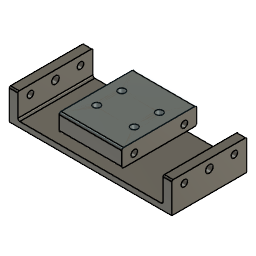
Sample Fixtures (Autodesk Fusion 360 archive; units mm, degrees)
design "Updated X stage"
part number: 2026-06-25-14-53-23-584
Autodesk Fusion 360 part; units mm, degrees
sketch "Sketch1" plane through (0, 0, 0) normal (0, 0, 1) x (1, 0, 0)
  line L0 (65, -30) -> (-65, -30)
  line L1 (-65, -30) -> (-65, 30)
  line L2 (-65, 30) -> (65, 30)
  line L3 (65, 30) -> (65, -30)
  line L4 (65, -30) -> (-65, 30) construction
  line L5 (-65, -30) -> (65, 30) construction
  line L6 (10, -15) -> (-10, -15) construction
  line L7 (-10, -15) -> (-10, 15) construction
  line L8 (-10, 15) -> (10, 15) construction
  line L9 (10, 15) -> (10, -15) construction
  line L10 (10, -15) -> (-10, 15) construction
  line L11 (-10, -15) -> (10, 15) construction
  circle A0 centre (10, 15) radius 2.05
  circle A1 centre (10, -15) radius 2.05
  circle A2 centre (-10, -15) radius 2.05
  circle A3 centre (-10, 15) radius 2.05
  dimension "d1" = 60
  dimension "d2" = 130
  dimension "d5" = 20
  dimension "d6" = 30
  dimension "d7" = 4.1
  constraint horizontal L0
  constraint perpendicular L0 L1
  constraint parallel L0 L2
  constraint parallel L1 L3
  constraint coincident L4 origin
  constraint coincident L5 origin
  constraint horizontal L6
  constraint perpendicular L6 L7
  constraint parallel L6 L8
  constraint parallel L7 L9
  constraint coincident L10 origin
  constraint coincident L11 origin
  constraint coincident L8.end L9.start
  constraint coincident L6.start L9.end
  constraint coincident L6.end L7.start
  constraint coincident L7.end L8.start
  constraint equal A0 A1
  constraint equal A1 A2
  constraint equal A2 A3
  measures "d1" distance of L0.start L2.end
  measures "d2" distance of L1.end L2.end
  measures "d5" distance of L7.end L8.end
  measures "d6" distance of L6.start L8.end
  measures "d7" diameter of A0
extrude "Extrude1" add sketch "Sketch1" along normal blind 4.5 makes body 1
sketch "Sketch2" plane through (0, 0, 4.5) normal (0, 0, 1) x (-1, 0, 0)
  circle A0 centre (10, 15) radius 2.05
  circle A1 centre (-10, 15) radius 2.05
  circle A2 centre (-10, -15) radius 2.05
  circle A3 centre (10, -15) radius 2.05
  line L0 (-65, -30) -> (65, -30)
  line L1 (65, -30) -> (65, 30)
  line L2 (65, 30) -> (-65, 30)
  line L3 (-65, 30) -> (-65, -30)
  line L4 (-10, 15) -> (10, 15) construction
  line L5 (10, 15) -> (10, -15) construction
  line L6 (10, -15) -> (-10, -15) construction
  line L7 (-10, -15) -> (-10, 15) construction
  line L8 (-10, 15) -> (10, -15) construction
  line L9 (10, 15) -> (-10, -15) construction
  circle A4 centre (-10, -15) radius 3.65
  circle A5 centre (-10, 15) radius 3.65
  circle A6 centre (10, 15) radius 3.65
  circle A7 centre (10, -15) radius 3.65
  dimension "d8" = 7.3
  constraint horizontal L4
  constraint perpendicular L4 L5
  constraint parallel L4 L6
  constraint parallel L5 L7
  constraint coincident L8 origin
  constraint coincident L9 origin
  constraint coincident A1.centre L4.start
  constraint concentric A2 A4
  constraint concentric A0 A6
  constraint concentric A3 A7
  constraint equal A4 A5
  constraint equal A5 A6
  constraint equal A6 A7
  measures "d8" diameter of A4
  measures "d27" diameter of origin
extrude "Extrude2" cut sketch "Sketch2" against normal blind 3.2 contours A4 | A5 | A6 | A7 bodies 1
sketch "Sketch3" plane through (0, 0, 4.5) normal (0, 0, 1) x (-1, 0, 0)
  line L0 (-65, -30) -> (65, -30)
  line L1 (65, -30) -> (65, 30)
  line L2 (65, 30) -> (-65, 30)
  line L3 (-65, 30) -> (-65, -30)
  circle A0 centre (10, -15) radius 3.65
  circle A1 centre (-10, -15) radius 3.65
  circle A2 centre (10, 15) radius 3.65
  circle A3 centre (-10, 15) radius 3.65
  line L4 (65, -30) -> (58, -30)
  line L5 (58, -30) -> (58, 30)
  line L6 (58, 30) -> (65, 30)
  line L7 (65, 30) -> (65, -30)
  line L8 (-65, -30) -> (-58, -30)
  line L9 (-58, -30) -> (-58, 30)
  line L10 (-58, 30) -> (-65, 30)
  line L11 (-65, 30) -> (-65, -30)
  dimension "d11" = 7
  dimension "d12" = 7
  constraint horizontal L4
  constraint vertical L5
  constraint horizontal L6
  constraint vertical L7
  constraint coincident L2 L5.end
  constraint coincident L0.end L1.start
  constraint horizontal L8
  constraint vertical L9
  constraint horizontal L10
  constraint vertical L11
  constraint coincident L2 L9.end
  constraint coincident L0.start L3.end
  measures "d11" distance of L5 L7
  measures "d12" distance of L9 L11
extrude "Extrude3" add sketch "Sketch3" along normal blind 20 contours L0 L2 L3 L8 L9 L10 L11 | L0 L1 L2 L4 L5 L6 L7 bodies 1
sketch "Sketch4" plane through (65, 0, 0) normal (1, 0, 0) x (0, 1, 0)
  line L0 (-30, 0) -> (30, 0)
  line L1 (30, 0) -> (30, 24.5)
  line L2 (30, 24.5) -> (-30, 24.5)
  line L3 (-30, 24.5) -> (-30, 0)
  line L4 (-30.1781, 17.5) -> (30.1781, 17.5) construction
  circle A0 centre (-20, 17.5) radius 2.575
  circle A1 centre (0, 17.5) radius 3
  circle A2 centre (20, 17.5) radius 2.575
  line L5 (30, 0) -> (-30, 0)
  line L6 (0, 24.5) -> (0, 0) construction
  dimension "d15" = 6
  dimension "d16" = 20
  dimension "d17" = 20
  dimension "d36" = 7
  dimension "d48" = 5.15
  constraint coincident L4 A0.centre
  constraint midpoint L4 A1.centre
  constraint coincident L4 A2.centre
  constraint midpoint L2 L6.start
  constraint coincident L6.end origin
  constraint coincident A1.centre L6
  constraint equal A0 A2
  measures "d15" diameter of A1
  measures "d16" distance of A1.centre A2.centre
  measures "d17" distance of A0.centre A1.centre
  measures "d36" distance of L2 L4
  measures "d48" diameter of A2
extrude "Extrude4" cut sketch "Sketch4" against normal through all contours A0 | A1 | A2 bodies 1
ref_plane "WorkPlane1" through (0, 0, 12.5) normal (0, 0, 1) x (1, 0, 0)
sketch "Sketch5" plane through (0, 0, 12.5) normal (0, 0, 1) x (1, 0, 0)
  line L0 (-25, 30) -> (25, 30)
  line L1 (25, 30) -> (25, -30)
  line L2 (25, -30) -> (-25, -30)
  line L3 (-25, -30) -> (-25, 30)
  line L4 (-25, 30) -> (25, -30) construction
  line L5 (25, 30) -> (-25, -30) construction
  line L6 (-65, 30) -> (65, 30)
  dimension "d22" = 50
  constraint horizontal L0
  constraint perpendicular L0 L1
  constraint parallel L0 L2
  constraint parallel L1 L3
  constraint coincident L4 origin
  constraint coincident L5 origin
  constraint collinear L0 L6
  measures "d22" distance of L1.end L2.end
extrude "Extrude5" add sketch "Sketch5" along normal blind 14 separate body makes body 2
sketch "Sketch6" plane through (0, 0, 26.5) normal (0, 0, 1) x (-1, 0, 0)
  line L0 (25, -30) -> (25, 30)
  line L1 (25, 30) -> (-25, 30)
  line L2 (-25, 30) -> (-25, -30)
  line L3 (-25, -30) -> (25, -30)
  line L4 (15, -10) -> (-15, -10) construction
  line L5 (-15, -10) -> (-15, 10) construction
  line L6 (-15, 10) -> (15, 10) construction
  line L7 (15, 10) -> (15, -10) construction
  line L8 (15, -10) -> (-15, 10) construction
  line L9 (-15, -10) -> (15, 10) construction
  circle A0 centre (-15, 10) radius 2.8
  circle A1 centre (15, 10) radius 2.8
  circle A2 centre (15, -10) radius 2.8
  circle A3 centre (-15, -10) radius 2.8
  dimension "d25" = 20
  dimension "d26" = 30
  dimension "d27" = 5.6
  constraint horizontal L4
  constraint perpendicular L4 L5
  constraint parallel L4 L6
  constraint parallel L5 L7
  constraint coincident L8 origin
  constraint coincident L9 origin
  constraint coincident L5.end L6.start
  constraint coincident L6.end L7.start
  constraint coincident L4.start L7.end
  constraint coincident L4.end L5.start
  constraint equal A0 A3
  constraint equal A0 A1
  constraint equal A1 A2
  measures "d25" distance of L4.end L5.end
  measures "d26" distance of L5.end L6.end
  measures "d27" diameter of A3
extrude "Extrude6" cut sketch "Sketch6" against normal up to surface (14 mm away) contours A0 | A1 | A2 | A3 bodies 2
sketch "Sketch7" plane through (25, 0, 0) normal (1, 0, 0) x (0, 1, 0)
  line L0 (30, 26.5) -> (-30, 26.5)
  line L1 (-30, 26.5) -> (-30, 12.5)
  line L2 (-30, 12.5) -> (30, 12.5)
  line L3 (30, 12.5) -> (30, 26.5)
  line L4 (-30, 18.3) -> (30, 18.3) construction
  circle A0 centre (-20, 18.3) radius 2.6
  circle A1 centre (0, 18.3) radius 3
  circle A2 centre (20, 18.3) radius 2.6
  dimension "d30" = 8.2
  dimension "d31" = 20
  dimension "d32" = 20
  dimension "d33" = 6
  dimension "d49" = 5.2
  constraint coincident L1 L4.start
  constraint coincident L3 L4.end
  constraint perpendicular L3 L4
  constraint coincident L4 A0.centre
  constraint midpoint L4 A1.centre
  constraint coincident L4 A2.centre
  constraint equal A0 A2
  measures "d30" distance of L0 L4
  measures "d31" distance of A1.centre A2.centre
  measures "d32" distance of A0.centre A1.centre
  measures "d33" diameter of A1
  measures "d49" diameter of A0
extrude "Extrude7" cut sketch "Sketch7" against normal up to surface (50 mm away) contours A0 | A2 bodies 2
sketch "Sketch8" plane through (65, 0, 0) normal (1, 0, 0) x (0, 1, 0)
  circle A0 centre (20, 17.5) radius 2.575
  circle A1 centre (-20, 17.5) radius 2.575
  circle A2 centre (0, 17.5) radius 3
  line L0 (-30, 0) -> (30, 0)
  line L1 (30, 0) -> (30, 24.5)
  line L2 (30, 24.5) -> (-30, 24.5)
  line L3 (-30, 24.5) -> (-30, 0)
  circle A3 centre (-20, 17.5) radius 2.95
  circle A4 centre (20, 17.5) radius 2.95
  dimension "d38" = 5.9
  constraint coincident A1.centre A3.centre
  constraint coincident A0.centre A4.centre
  constraint equal A3 A4
  measures "d38" diameter of A4
extrude "Extrude8" add sketch "Sketch8" against normal up to surface (130 mm away) separate body contours A0 | A1 | A3 | A4 makes body 3 at (21.6667, 22.9353, 17.2063) makes body 4 at (-21.6667, -17.0537, 17.353)
sketch "Sketch9" plane through (0, 0, 26.5) normal (0, 0, 1) x (-1, 0, 0)
  circle A0 centre (-15, -10) radius 2.8
  circle A1 centre (15, -10) radius 2.8
  circle A2 centre (-15, 10) radius 2.8
  circle A3 centre (15, 10) radius 2.8
  line L0 (25, 30) -> (-25, 30)
  line L1 (-25, 30) -> (-25, -30)
  line L2 (-25, -30) -> (25, -30)
  line L3 (25, -30) -> (25, 30)
split "Split1" by plane through (0, 0, 0) normal (1, 0, 0) bodies 3 makes body 5 at (21.6667, 22.9353, 17.2063)
sketch "Sketch10" plane through (0, 0, 0) normal (1, 0, 0) x (0, 1, 0)
  circle A0 centre (20, 17.5) radius 2.95
  circle A1 centre (20, 17.5) radius 1.25
  dimension "d42" = 2.5
  constraint concentric A0 A1
  measures "d42" diameter of A1
extrude "Extrude9" add sketch "Sketch10" along normal blind 4 contours A1 bodies 3
sketch "Sketch11" plane through (0, 0, 0) normal (-1, 0, 0) x (0, -1, 0)
  circle A0 centre (-20, 17.5) radius 2.95
  circle A1 centre (-20, 17.5) radius 1.325
  dimension "d45" = 2.65
  constraint concentric A0 A1
  measures "d45" diameter of A1
extrude "Extrude10" cut sketch "Sketch11" against normal blind 4 contours A1 bodies 5
sketch "Sketch12" plane through (0, 0, 0) normal (0, 1, 0) x (1, 0, 0)
fillet "Fillet1" radius 1 4 edges at (-61.5, 30, 24.5) (61.5, 30, 24.5) (61.5, -30, 24.5) (-61.5, -30, 24.5) on bodies 1
fillet "Fillet2" radius 1.5 2 edges at (-58, 0, 4.5) (58, 0, 4.5) on bodies 1
fillet "Fillet3" radius 1.5 2 edges at (0, -30, 12.5) (0, 30, 12.5) on bodies 2
fillet "Fillet3" radius 1.5 2 edges at (0, 30, 26.5) (0, -30, 26.5) on bodies 2
delete_body "RemoveBody1" bodies 3
delete_body "RemoveBody2" bodies 4
delete_body "RemoveBody3" bodies 5
named bodies: "Ystage", "Y mount", "Male Support rod", "Support rod (1)"

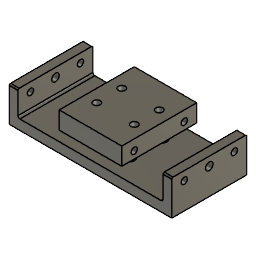
design "Updated Y stage"
part number: 2026-06-25-14-53-23-584
Autodesk Fusion 360 part; units mm, degrees
sketch "Sketch1" plane through (0, 0, 0) normal (0, 0, 1) x (1, 0, 0)
  line L0 (65, -30) -> (-65, -30)
  line L1 (-65, -30) -> (-65, 30)
  line L2 (-65, 30) -> (65, 30)
  line L3 (65, 30) -> (65, -30)
  line L4 (65, -30) -> (-65, 30) construction
  line L5 (-65, -30) -> (65, 30) construction
  line L6 (13, -13) -> (-13, -13) construction
  line L7 (-13, -13) -> (-13, 13) construction
  line L8 (-13, 13) -> (13, 13) construction
  line L9 (13, 13) -> (13, -13) construction
  line L10 (13, -13) -> (-13, 13) construction
  line L11 (-13, -13) -> (13, 13) construction
  circle A0 centre (13, 13) radius 3
  circle A1 centre (13, -13) radius 3
  circle A2 centre (-13, -13) radius 3
  circle A3 centre (-13, 13) radius 3
  dimension "d1" = 60
  dimension "d2" = 130
  dimension "d5" = 26
  dimension "d6" = 26
  dimension "d7" = 6
  constraint horizontal L0
  constraint perpendicular L0 L1
  constraint parallel L0 L2
  constraint parallel L1 L3
  constraint coincident L4 origin
  constraint coincident L5 origin
  constraint horizontal L6
  constraint perpendicular L6 L7
  constraint parallel L6 L8
  constraint parallel L7 L9
  constraint coincident L10 origin
  constraint coincident L11 origin
  constraint coincident L8.end L9.start
  constraint coincident L6.start L9.end
  constraint coincident L6.end L7.start
  constraint coincident L7.end L8.start
  constraint equal A0 A1
  constraint equal A1 A2
  constraint equal A2 A3
  measures "d1" distance of L0.start L2.end
  measures "d2" distance of L1.end L2.end
  measures "d5" distance of L7.end L8.end
  measures "d6" distance of L6.start L8.end
  measures "d7" diameter of A0
extrude "Extrude1" add sketch "Sketch1" along normal blind 8 makes body 1
sketch "Sketch2" plane through (0, 0, 8) normal (0, 0, 1) x (-1, 0, 0)
  circle A0 centre (13, 13) radius 3
  circle A1 centre (-13, 13) radius 3
  circle A2 centre (-13, -13) radius 3
  circle A3 centre (13, -13) radius 3
  line L0 (-65, -30) -> (65, -30)
  line L1 (65, -30) -> (65, 30)
  line L2 (65, 30) -> (-65, 30)
  line L3 (-65, 30) -> (-65, -30)
  line L4 (-13, 13) -> (13, 13) construction
  line L5 (13, 13) -> (13, -13) construction
  line L6 (13, -13) -> (-13, -13) construction
  line L7 (-13, -13) -> (-13, 13) construction
  line L8 (-13, 13) -> (13, -13) construction
  line L9 (13, 13) -> (-13, -13) construction
  circle A4 centre (-13, -13) radius 5.15
  circle A5 centre (-13, 13) radius 5.15
  circle A6 centre (13, 13) radius 5.15
  circle A7 centre (13, -13) radius 5.15
  dimension "d8" = 10.3
  constraint horizontal L4
  constraint perpendicular L4 L5
  constraint parallel L4 L6
  constraint parallel L5 L7
  constraint coincident L8 origin
  constraint coincident L9 origin
  constraint coincident A1.centre L4.start
  constraint concentric A2 A4
  constraint concentric A0 A6
  constraint concentric A3 A7
  constraint equal A4 A5
  constraint equal A5 A6
  constraint equal A6 A7
  measures "d8" diameter of A4
  measures "d27" diameter of origin
extrude "Extrude2" cut sketch "Sketch2" against normal blind 6.1 contours A4 | A5 | A6 | A7 bodies 1
sketch "Sketch3" plane through (0, 0, 8) normal (0, 0, 1) x (-1, 0, 0)
  line L0 (-65, -30) -> (65, -30)
  line L1 (65, -30) -> (65, 30)
  line L2 (65, 30) -> (-65, 30)
  line L3 (-65, 30) -> (-65, -30)
  circle A0 centre (13, -13) radius 5.15
  circle A1 centre (-13, -13) radius 5.15
  circle A2 centre (13, 13) radius 5.15
  circle A3 centre (-13, 13) radius 5.15
  line L4 (65, -30) -> (58, -30)
  line L5 (58, -30) -> (58, 30)
  line L6 (58, 30) -> (65, 30)
  line L7 (65, 30) -> (65, -30)
  line L8 (-65, -30) -> (-58, -30)
  line L9 (-58, -30) -> (-58, 30)
  line L10 (-58, 30) -> (-65, 30)
  line L11 (-65, 30) -> (-65, -30)
  dimension "d11" = 7
  dimension "d12" = 7
  constraint horizontal L4
  constraint vertical L5
  constraint horizontal L6
  constraint vertical L7
  constraint coincident L2 L5.end
  constraint coincident L0.end L1.start
  constraint horizontal L8
  constraint vertical L9
  constraint horizontal L10
  constraint vertical L11
  constraint coincident L2 L9.end
  constraint coincident L0.start L3.end
  measures "d11" distance of L5 L7
  measures "d12" distance of L9 L11
extrude "Extrude3" add sketch "Sketch3" along normal blind 20 contours L0 L2 L3 L8 L9 L10 L11 | L0 L1 L2 L4 L5 L6 L7 bodies 1
sketch "Sketch4" plane through (65, 0, 0) normal (1, 0, 0) x (0, 1, 0)
  line L0 (-30, 0) -> (30, 0)
  line L1 (30, 0) -> (30, 28)
  line L2 (30, 28) -> (-30, 28)
  line L3 (-30, 28) -> (-30, 0)
  line L4 (-30.1781, 21) -> (30.1781, 21) construction
  circle A0 centre (-20, 21) radius 2.5
  circle A1 centre (0, 21) radius 3
  circle A2 centre (20, 21) radius 2.5
  line L5 (30, 0) -> (-30, 0)
  line L6 (0, 28) -> (0, 0) construction
  dimension "d15" = 6
  dimension "d16" = 20
  dimension "d17" = 20
  dimension "d36" = 7
  dimension "d48" = 5
  constraint coincident L4 A0.centre
  constraint midpoint L4 A1.centre
  constraint coincident L4 A2.centre
  constraint midpoint L2 L6.start
  constraint coincident L6.end origin
  constraint coincident A1.centre L6
  constraint equal A0 A2
  measures "d15" diameter of A1
  measures "d16" distance of A1.centre A2.centre
  measures "d17" distance of A0.centre A1.centre
  measures "d36" distance of L2 L4
  measures "d48" diameter of A2
extrude "Extrude4" cut sketch "Sketch4" against normal through all contours A0 | A1 | A2 bodies 1
ref_plane "WorkPlane1" through (0, 0, 16) normal (0, 0, 1) x (1, 0, 0)
sketch "Sketch5" plane through (0, 0, 16) normal (0, 0, 1) x (1, 0, 0)
  line L0 (-25, 30) -> (25, 30)
  line L1 (25, 30) -> (25, -30)
  line L2 (25, -30) -> (-25, -30)
  line L3 (-25, -30) -> (-25, 30)
  line L4 (-25, 30) -> (25, -30) construction
  line L5 (25, 30) -> (-25, -30) construction
  line L6 (-65, 30) -> (65, 30)
  dimension "d22" = 50
  constraint horizontal L0
  constraint perpendicular L0 L1
  constraint parallel L0 L2
  constraint parallel L1 L3
  constraint coincident L4 origin
  constraint coincident L5 origin
  constraint collinear L0 L6
  measures "d22" distance of L1.end L2.end
extrude "Extrude5" add sketch "Sketch5" along normal blind 14 separate body makes body 2
sketch "Sketch6" plane through (0, 0, 30) normal (0, 0, 1) x (-1, 0, 0)
  line L0 (25, -30) -> (25, 30)
  line L1 (25, 30) -> (-25, 30)
  line L2 (-25, 30) -> (-25, -30)
  line L3 (-25, -30) -> (25, -30)
  line L4 (15, -10) -> (-15, -10) construction
  line L5 (-15, -10) -> (-15, 10) construction
  line L6 (-15, 10) -> (15, 10) construction
  line L7 (15, 10) -> (15, -10) construction
  line L8 (15, -10) -> (-15, 10) construction
  line L9 (-15, -10) -> (15, 10) construction
  circle A0 centre (-15, 10) radius 2.8
  circle A1 centre (15, 10) radius 2.8
  circle A2 centre (15, -10) radius 2.8
  circle A3 centre (-15, -10) radius 2.8
  dimension "d25" = 20
  dimension "d26" = 30
  dimension "d27" = 5.6
  constraint horizontal L4
  constraint perpendicular L4 L5
  constraint parallel L4 L6
  constraint parallel L5 L7
  constraint coincident L8 origin
  constraint coincident L9 origin
  constraint coincident L5.end L6.start
  constraint coincident L6.end L7.start
  constraint coincident L4.start L7.end
  constraint coincident L4.end L5.start
  constraint equal A0 A3
  constraint equal A0 A1
  constraint equal A1 A2
  measures "d25" distance of L4.end L5.end
  measures "d26" distance of L5.end L6.end
  measures "d27" diameter of A3
extrude "Extrude6" cut sketch "Sketch6" against normal up to surface (14 mm away) contours A0 | A1 | A2 | A3 bodies 2
sketch "Sketch7" plane through (25, 0, 0) normal (1, 0, 0) x (0, 1, 0)
  line L0 (30, 30) -> (-30, 30)
  line L1 (-30, 30) -> (-30, 16)
  line L2 (-30, 16) -> (30, 16)
  line L3 (30, 16) -> (30, 30)
  line L4 (-30, 21.8) -> (30, 21.8) construction
  circle A0 centre (-20, 21.8) radius 2.5
  circle A1 centre (0, 21.8) radius 3
  circle A2 centre (20, 21.8) radius 2.5
  dimension "d30" = 8.2
  dimension "d31" = 20
  dimension "d32" = 20
  dimension "d33" = 6
  dimension "d49" = 5
  constraint coincident L1 L4.start
  constraint coincident L3 L4.end
  constraint perpendicular L3 L4
  constraint coincident L4 A0.centre
  constraint midpoint L4 A1.centre
  constraint coincident L4 A2.centre
  constraint equal A0 A2
  measures "d30" distance of L0 L4
  measures "d31" distance of A1.centre A2.centre
  measures "d32" distance of A0.centre A1.centre
  measures "d33" diameter of A1
  measures "d49" diameter of A0
extrude "Extrude7" cut sketch "Sketch7" against normal up to surface (50 mm away) contours A0 | A2 bodies 2
sketch "Sketch8" plane through (65, 0, 0) normal (1, 0, 0) x (0, 1, 0)
  circle A0 centre (20, 21) radius 2.5
  circle A1 centre (-20, 21) radius 2.5
  circle A2 centre (0, 21) radius 3
  line L0 (-30, 0) -> (30, 0)
  line L1 (30, 0) -> (30, 28)
  line L2 (30, 28) -> (-30, 28)
  line L3 (-30, 28) -> (-30, 0)
  circle A3 centre (-20, 21) radius 2.95
  circle A4 centre (20, 21) radius 2.95
  dimension "d38" = 5.9
  constraint coincident A1.centre A3.centre
  constraint coincident A0.centre A4.centre
  constraint equal A3 A4
  measures "d38" diameter of A4
extrude "Extrude8" add sketch "Sketch8" against normal up to surface (130 mm away) separate body contours A0 | A1 | A3 | A4 makes body 3 at (21.6667, 22.9353, 20.7063) makes body 4 at (-21.6667, -17.0537, 20.853)
sketch "Sketch9" plane through (0, 0, 30) normal (0, 0, 1) x (-1, 0, 0)
  circle A0 centre (-15, -10) radius 2.8
  circle A1 centre (15, -10) radius 2.8
  circle A2 centre (-15, 10) radius 2.8
  circle A3 centre (15, 10) radius 2.8
  line L0 (25, 30) -> (-25, 30)
  line L1 (-25, 30) -> (-25, -30)
  line L2 (-25, -30) -> (25, -30)
  line L3 (25, -30) -> (25, 30)
split "Split1" by plane through (0, 0, 0) normal (1, 0, 0) bodies 3 makes body 5 at (21.6667, 22.9353, 20.7063)
sketch "Sketch10" plane through (0, 0, 0) normal (1, 0, 0) x (0, 1, 0)
  circle A0 centre (20, 21) radius 2.95
  circle A1 centre (20, 21) radius 1.25
  dimension "d42" = 2.5
  constraint concentric A0 A1
  measures "d42" diameter of A1
extrude "Extrude9" add sketch "Sketch10" along normal blind 4 contours A1 bodies 3
sketch "Sketch11" plane through (0, 0, 0) normal (-1, 0, 0) x (0, -1, 0)
  circle A0 centre (-20, 21) radius 2.95
  circle A1 centre (-20, 21) radius 1.325
  dimension "d45" = 2.65
  constraint concentric A0 A1
  measures "d45" diameter of A1
extrude "Extrude10" cut sketch "Sketch11" against normal blind 4 contours A1 bodies 5
sketch "Sketch12" plane through (0, 0, 0) normal (0, 1, 0) x (1, 0, 0)
fillet "Fillet1" radius 1 4 edges at (-61.5, 30, 28) (61.5, 30, 28) (61.5, -30, 28) (-61.5, -30, 28) on bodies 1
fillet "Fillet2" radius 1.5 2 edges at (-58, 0, 8) (58, 0, 8) on bodies 1
delete_body "RemoveBody1" bodies 3
delete_body "RemoveBody2" bodies 4
delete_body "RemoveBody3" bodies 5
named bodies: "Ystage", "Y mount", "Male Support rod", "Support rod (1)"

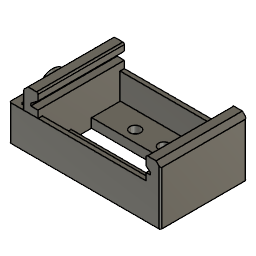
design "New PCB Holder"
part number: 2026-06-14-23-15-08-498
Autodesk Fusion 360 part; units mm, degrees
sketch "Sketch1" plane through (0, 0, 0) normal (0, 0, 1) x (1, 0, 0)
  line L0 (0, 0) -> (105, 0)
  line L1 (105, 0) -> (105, 60)
  line L2 (105, 60) -> (0, 60)
  line L3 (0, 60) -> (0, 0)
  dimension "d1" = 105
  dimension "d2" = 60
  constraint horizontal L0
  constraint vertical L1
  constraint horizontal L2
  constraint vertical L3
  constraint coincident L0.start L3.end
  measures "d1" distance of L1.end L2.end
  measures "d2" distance of L0.end L1.end
extrude "Extrude1" add sketch "Sketch1" along normal blind 6.5 makes body 1
sketch "Sketch2" plane through (0, 0, 6.5) normal (0, 0, 1) x (-1, 0, 0)
  line L0 (0, -60) -> (0, 0)
  line L1 (0, 0) -> (-105, 0)
  line L2 (-105, 0) -> (-105, -60)
  line L3 (-105, -60) -> (0, -60)
  line L4 (0, -30) -> (-105, -30) construction
  line L5 (-52.5, -60) -> (-52.5, 0) construction
  line L6 (-62.5, -15) -> (-42.5, -15) construction
  line L7 (-42.5, -15) -> (-42.5, -45) construction
  line L8 (-42.5, -45) -> (-62.5, -45) construction
  line L9 (-62.5, -45) -> (-62.5, -15) construction
  line L10 (-62.5, -15) -> (-42.5, -45) construction
  line L11 (-42.5, -15) -> (-62.5, -45) construction
  circle A0 centre (-42.5, -45) radius 2.025
  circle A1 centre (-42.5, -15) radius 2.025
  circle A2 centre (-62.5, -15) radius 2.025
  circle A3 centre (-62.5, -45) radius 2.025
  circle A4 centre (-42.5, -15) radius 3.75 construction
  circle A5 centre (-42.5, -45) radius 3.75 construction
  point P0 (-52.5, -30)
  dimension "d56" = 20
  dimension "d57" = 30
  dimension "d58" = 4.05
  dimension "d63" = 7.5
  dimension "d64" = 7.5
  constraint midpoint L0 L4.start
  constraint midpoint L2 L4.end
  constraint midpoint L3 L5.start
  constraint midpoint L1 L5.end
  constraint horizontal L6
  constraint perpendicular L6 L7
  constraint parallel L6 L8
  constraint parallel L7 L9
  constraint coincident L10 P0
  constraint coincident L11 P0
  constraint coincident L7.end L8.start
  constraint coincident L6.end L7.start
  constraint coincident L6.start L9.end
  constraint coincident L8.end L9.start
  constraint equal A2 A3
  constraint equal A1 A2
  constraint equal A0 A1
  constraint concentric A1 A4
  constraint concentric A0 A5
  constraint coincident L4 P0
  constraint coincident L5 P0
  measures "d56" distance of L7.end L8.end
  measures "d57" distance of L6.start L8.end
  measures "d58" diameter of A3
  measures "d63" diameter of A4
  measures "d64" diameter of A5
extrude "Extrude2" cut sketch "Sketch2" against normal through all contours A0 | A1 | A2 | A3 bodies 1
sketch "Sketch11" plane through (0, 0, 6.5) normal (0, 0, 1) x (-1, 0, 0)
  circle A0 centre (-42.5, -45) radius 3.75
  circle A1 centre (-62.5, -45) radius 3.75
  circle A2 centre (-62.5, -15) radius 3.75
  circle A3 centre (-42.5, -15) radius 3.75
  line L0 (-42.5, -15) -> (-62.5, -45) construction
  line L1 (-42.5, -15) -> (-42.5, -45) construction
  line L2 (-62.5, -15) -> (-42.5, -45) construction
  line L3 (-42.5, -45) -> (-62.5, -45) construction
  line L4 (-62.5, -45) -> (-62.5, -15) construction
  line L5 (-62.5, -15) -> (-42.5, -15) construction
  circle A4 centre (-62.5, -15) radius 2.025
  circle A5 centre (-62.5, -45) radius 2.025
  circle A6 centre (-42.5, -45) radius 2.025
  circle A7 centre (-42.5, -15) radius 2.025
  circle A8 centre (-62.5, -15) radius 2.025
  circle A9 centre (-62.5, -45) radius 2.025
  circle A10 centre (-42.5, -45) radius 2.025
  constraint equal A0 A3
  constraint equal A0 A1
  constraint equal A1 A2
  constraint coincident A0.centre L1
  constraint coincident A2.centre L2
  constraint coincident A0.centre L3
  constraint coincident A1.centre L4
  constraint coincident A1.centre L3
  constraint coincident A2.centre L5
  constraint coincident A2.centre L2.start
  constraint coincident A1.centre L0.end
  constraint coincident A0.centre L1.end
  constraint concentric A3 A7
  constraint equal A4 A8
  constraint equal A5 A8
  constraint equal A6 A9
  constraint equal A7 A10
extrude "Extrude11" cut sketch "Sketch11" against normal blind 5 bodies 1
sketch "Sketch3" plane through (0, 0, 6.5) normal (0, 0, 1) x (-1, 0, 0)
  line L0 (0, -60) -> (0, 0)
  line L1 (0, 0) -> (-105, 0)
  line L2 (-105, 0) -> (-105, -60)
  line L3 (-105, -60) -> (0, -60)
  line L4 (-105, -57) -> (-5, -57)
  line L5 (-5, -57) -> (-5, -3)
  line L6 (-5, -3) -> (-105, -3)
  circle A0 centre (-62.5, -45) radius 3.75
  circle A1 centre (-62.5, -15) radius 3.75
  circle A2 centre (-42.5, -45) radius 3.75
  circle A3 centre (-42.5, -15) radius 3.75
  dimension "d11" = 3
  dimension "d12" = 3
  dimension "d13" = 5
  constraint coincident L2 L4.start
  constraint perpendicular L2 L4
  constraint perpendicular L4 L5
  constraint coincident L2 L6.end
  constraint perpendicular L2 L6
  measures "d11" distance of L3 L4
  measures "d12" distance of L1 L6
  measures "d13" distance of L0 L5
extrude "Extrude3" add sketch "Sketch3" along normal blind 18 contours L0 L1 L2 L3 L4 L5 L6 bodies 1
ref_plane "WorkPlane1" through (20, 0, 0) normal (1, 0, 0) x (0, 1, 0)
sketch "Sketch4" plane through (20, 0, 0) normal (1, 0, 0) x (0, 1, 0)
  line L0 (3.15, 6.3) -> (56.85, 6.3)
  line L1 (56.85, 6.3) -> (56.85, 24.5)
  line L2 (60, 40) -> (0, 40)
  line L3 (0, 24.5) -> (3.15, 24.5)
  line L4 (3.15, 24.5) -> (3.15, 6.3)
  line L5 (60, 40) -> (60, 24.5)
  line L6 (60, 24.5) -> (56.85, 24.5)
  line L7 (0, 0) -> (60, 0)
  line L8 (3, 6.5) -> (3, 24.5)
  line L9 (57, 6.5) -> (57, 24.5)
  line L10 (0, 40) -> (0, 24.5)
  line L11 (0, 0) -> (0, 24.5)
  line L12 (60, 0) -> (60, 24.5)
  line L13 (23.025, 6.3) -> (36.975, 6.3)
  line L14 (30, 0) -> (30, 6.3) construction
  line L15 (23.025, 6.3) -> (36.975, 6.3)
  line L16 (36.975, 6.3) -> (36.975, 0)
  line L17 (36.975, 0) -> (23.025, 0)
  line L18 (23.025, 0) -> (23.025, 6.3)
  line L19 (3, 6.5) -> (57, 6.5)
  dimension "d25" = 15.5
  dimension "d78" = 0.15
  dimension "d79" = 0.15
  dimension "d103" = 0.2
  dimension "d121" = 13.95
  dimension "d122" = 6.975
  constraint horizontal L0
  constraint perpendicular L0 L1
  constraint perpendicular L1 L2
  constraint perpendicular L0 L4
  constraint perpendicular L2 L5
  constraint perpendicular L1 L6
  constraint horizontal L3
  constraint perpendicular L3 L10
  constraint collinear L10 L11
  constraint collinear L5 L12
  constraint equal L5 L10
  constraint horizontal L13
  constraint coincident L0 L13.start
  constraint midpoint L13 L14.end
  constraint midpoint L0 L14.end
  constraint coincident L5.end L6.start
  constraint horizontal L15
  constraint vertical L16
  constraint horizontal L17
  constraint vertical L18
  constraint collinear L7 L17
  constraint midpoint L7 L14.start
  measures "d25" distance of L2.start L5.end
  measures "d78" distance of L4 L8
  measures "d79" distance of L1 L9
  measures "d103" distance of L0 L19
  measures "d121" distance of L16.end L17.end
  measures "d122" distance of L14 L18
extrude "Extrude4" add sketch "Sketch4" against normal blind 10 separate body contours L0 L1 L4 L13 L15 L19 | L0 L7 L13 L15 L16 L17 L18 | L1 L2 L3 L4 L5 L6 L10 L19 makes body 2
sketch "Sketch5" plane through (105, 0, 0) normal (1, 0, 0) x (0, 1, 0)
  line L0 (0, 0) -> (60, 0)
  line L1 (60, 0) -> (60, 24.5)
  line L2 (60, 24.5) -> (57, 24.5)
  line L3 (57, 24.5) -> (57, 6.5)
  line L4 (57, 6.5) -> (3, 6.5)
  line L5 (3, 6.5) -> (3, 24.5)
  line L6 (3, 24.5) -> (0, 24.5)
  line L7 (0, 24.5) -> (0, 0)
  line L8 (0, 0) -> (60, 0)
  line L9 (60, 0) -> (60, 40)
  line L10 (60, 40) -> (0, 40)
  line L11 (0, 40) -> (0, 0)
  line L12 (60, 40) -> (0, 40)
  constraint horizontal L8
  constraint vertical L9
  constraint horizontal L10
  constraint vertical L11
  constraint coincident L0.start L7.end
  constraint collinear L1 L9
  constraint collinear L10 L12
extrude "Extrude5" add sketch "Sketch5" against normal blind 10 bodies 1
sketch "Sketch6" plane through (0, 0, 0) normal (0, -1, 0) x (1, 0, 0)
  line L0 (70, 18) -> (0, 18)
  line L1 (0, 18) -> (0, 0)
  line L2 (0, 0) -> (80, 0)
  line L3 (80, 0) -> (80, 25)
  line L4 (80, 25) -> (70, 25)
  line L5 (70, 25) -> (70, 18)
  line L6 (15, 31.15) -> (98, 31.15)
  line L7 (98, 31.15) -> (98, 29.5)
  line L8 (98, 29.5) -> (15, 29.5)
  line L9 (15, 29.5) -> (15, 31.15)
  line L10 (13.5, 18) -> (20, 18)
  line L11 (0, 18) -> (110, 18)
  line L12 (95, 24.5) -> (0, 24.5)
  line L13 (0, 24.5) -> (0, 0)
  line L14 (0, 0) -> (105, 0)
  line L15 (105, 0) -> (105, 40)
  line L16 (105, 40) -> (95, 40)
  line L17 (95, 40) -> (95, 24.5)
  line L18 (10, 24.5) -> (10, 40)
  line L19 (98, 31.15) -> (95, 33.4)
  line L20 (15, 31.15) -> (20, 34.9)
  line L21 (20, 40) -> (20, 24.5)
  dimension "d86" = 5
  dimension "d94" = 1.65
  dimension "d102" = 7
  dimension "d123" = 5
  dimension "d126" = 36.87
  dimension "d127" = 36.87
  constraint horizontal L6
  constraint vertical L7
  constraint horizontal L8
  constraint vertical L9
  constraint coincident L7.end L8.start
  constraint coincident L17 L19.end
  constraint coincident L20.end L21
  measures "d86" distance of L9 L18
  measures "d94" distance of L6.start L8.end
  measures "d102" distance of L7 L15
  measures "d123" distance of L8 L12
  measures "d126" angle of L6 L19
  measures "d127" angle of L6 L20
extrude "Extrude6" cut sketch "Sketch6" against normal up to surface (60 mm away) contours L6 L8 L17 L21 | L6 L8 L9 L21 | L6 L7 L8 L17 | L6 L20 L21 | L6 L17 L19 bodies 2
extrude "Extrude7" cut sketch "Sketch6" against normal up to surface (60 mm away) contours L6 L8 L17 L21 | L6 L8 L9 L21 | L6 L7 L8 L17 bodies 1
sketch "Sketch7" plane through (0, 0, 0) normal (-1, 0, 0) x (0, -1, 0)
  line L0 (-60, 0) -> (0, 0)
  line L1 (0, 0) -> (0, 24.5)
  line L2 (0, 24.5) -> (-60, 24.5)
  line L3 (-60, 24.5) -> (-60, 0)
  line L4 (0, 0) -> (-60, 0)
  line L5 (-60, 0) -> (-60, 24.5)
  line L6 (-60, 24.5) -> (0, 24.5)
  line L7 (0, 24.5) -> (0, 0)
  line L8 (0, 0) -> (-60, 24.5) construction
  line L9 (-60, 0) -> (0, 24.5) construction
  circle A0 centre (-30, 18.25) radius 2.95
  point P0 (-30, 12.25)
  dimension "d133" = 5.9
  dimension "d134" = 6
  constraint horizontal L4
  constraint perpendicular L4 L5
  constraint parallel L4 L6
  constraint parallel L5 L7
  constraint coincident L8 P0
  constraint coincident L9 P0
  constraint coincident L0.end L1.start
  constraint coincident L1.end L2.start
  constraint coincident L0.start L3.end
  constraint vertical P0 A0.centre
  measures "d133" diameter of A0
  measures "d134" distance of P0 A0.centre
extrude "Extrude8" cut sketch "Sketch7" against normal up to surface (5 mm away) contours A0 bodies 1
sketch "Sketch8" plane through (0, 0, 0) normal (0, -1, 0) x (1, 0, 0)
  line L0 (95, 24.5) -> (0, 24.5)
  line L1 (0, 24.5) -> (0, 0)
  line L2 (0, 0) -> (105, 0)
  line L3 (105, 0) -> (105, 40)
  line L4 (98, 29.5) -> (95, 29.5)
  line L5 (95, 29.5) -> (95, 24.5)
  line L6 (105, 40) -> (95, 40)
  line L7 (95, 31.15) -> (98, 31.15)
  line L8 (98, 31.15) -> (98, 29.5)
  line L9 (95, 40) -> (95, 31.15)
chamfer "Chamfer1" distance 3 angle 45 2 edges at (10, 30, 40) (105, 30, 40) tangent chain off on bodies 1 2
thread "Thread3" [suppressed]
fillet "Fillet1" radius 1 4 edges at (0, 0, 12.25) (0, 60, 12.25) (105, 60, 18.5) (105, 0, 18.5) on bodies 1
fillet "Fillet2" radius 1 2 edges at (5, 3, 15.5) (5, 57, 15.5) on bodies 1
thread "Thread7" [suppressed]
sketch "Sketch10" plane through (0, 0, 6.5) normal (0, 0, 1) x (-1, 0, 0)
  line L0 (-5, -37.1) -> (-95, -37.1)
  line L1 (-95, -37.1) -> (-95, -22.9)
  line L2 (-95, -22.9) -> (-5, -22.9)
  line L3 (-5, -22.9) -> (-5, -37.1)
  line L4 (-5, -37.1) -> (-95, -22.9) construction
  line L5 (-95, -37.1) -> (-5, -22.9) construction
  line L6 (0, -30) -> (-105, -30)
  line L7 (-95, -37.1) -> (-95, -22.9)
  line L8 (-95, 0) -> (-95, -60)
  line L9 (-5, -56) -> (-5, -4)
  point P0 (-50, -30)
  dimension "d91" = 14.2
  constraint horizontal L0
  constraint perpendicular L0 L1
  constraint parallel L0 L2
  constraint parallel L1 L3
  constraint coincident L4 P0
  constraint coincident L5 P0
  constraint coincident P0 L6
  constraint coincident L0.end L8
  constraint collinear L3 L9
  measures "d91" distance of L0 L2
extrude "Extrude10" cut sketch "Sketch10" against normal through all bodies 1
extrude "Extrude14" cut sketch "Sketch6" against normal through all contours L6 L17 L19 bodies 1
sketch "Sketch14" plane through (0, 0, 0) normal (-1, 0, 0) x (0, -1, 0)
  line L0 (-59, 24.5) -> (-59, 0)
  line L1 (-59, 0) -> (-1, 0)
  line L2 (-1, 0) -> (-1, 24.5)
  line L3 (-1, 24.5) -> (-59, 24.5)
  circle A0 centre (-30, 19.5) radius 10
  circle A1 centre (-30, 18.25) radius 2.95
  dimension "d129" = 20
  dimension "d130" = 5
  constraint vertical A0.centre A1.centre
  measures "d129" diameter of A0
  measures "d130" distance of L3 A0.centre
extrude "Extrude15" add sketch "Sketch14" against normal up to surface (5 mm away) contours L3 A0 picked at (-27.7328, 25.2768) bodies 1
fillet "Fillet3" radius 1 2 edges at (95, 30, 40) (20, 30, 40) on bodies 1 2
fillet "Fillet4" radius 1 2 edges at (2.5, 21.3397, 24.5) (2.5, 38.6603, 24.5) on bodies 1
named bodies: "Main pcb holder", "Adjuster"
